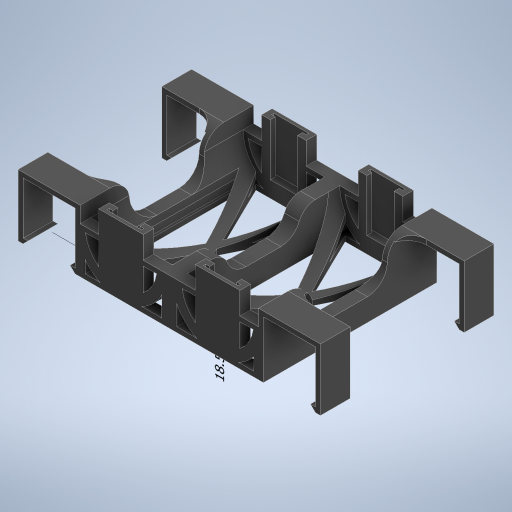
# Autodesk Inventor part: 電池ボックス
Saved by Autodesk Inventor 2024.1 (Build 281209000, 209)
## iProperties
Created: 2024-11-06
Part Number: 電池ボックス
Material: 一般
Document SubType Name: Modeling
Designer: hibik
Density: 1 g/cm^3
Appearance: 既定
Author: hibik
Autodesk Inventor part; units mm, degrees
ref_plane "YZ Plane" through (0, 0, 0) normal (1, 0, 0) x (0, 1, 0)
ref_plane "XZ Plane" through (0, 0, 0) normal (0, 1, 0) x (-1, 0, 0)
ref_plane "XY Plane" through (0, 0, 0) normal (0, 0, 1) x (1, 0, 0)
sketch "スケッチ1" plane through (0, 0, 0) normal (0, 0, 1) x (1, 0, 0)
  line L0 (-59, 0) -> (-38, 0)
  line L1 (-38, 0) -> (-38, -21)
  line L2 (-38, -21) -> (-59, -21)
  line L3 (-59, -21) -> (-59, 0)
  line L4 (-61, 2) -> (-36, 2)
  line L5 (-36, 2) -> (-36, -23)
  line L6 (-36, -23) -> (-61, -23)
  line L7 (-61, -23) -> (-61, 2)
  line L8 (-61, -23) -> (0, -23)
  line L9 (0, -23) -> (0, -21)
  line L10 (0, -21) -> (-61, -21)
  line L11 (-61, -21) -> (-61, -23)
  line L12 (-59, -23) -> (-57, -21)
  line L13 (-38, -23) -> (-40, -21)
  point P0 (0, 0)
  point P1 (-61, -10.5)
  point P2 (-59, -10.5)
  point P3 (-48.5, 2)
  point P4 (-48.5, 0)
  point P5 (-36, -21)
  dimension "d0" = 21
  dimension "d1" = 21
  dimension "d4" = 38
  dimension "d5" = 25
  dimension "d6" = 2
  dimension "d74" = 2
  dimension "d75" = 2
  constraints: 28 end point, 8 point on line, 6 parallel, 4 midpoint, 4 perpendicular, 3 horizontal, 1 horizontal alignment, 1 vertical alignment
  measures "d0" distance of L1.end L2.end
  measures "d1" distance of L0.end L1.end
  measures "d4" distance from line of point (0, 0) L1
  measures "d5" distance of L4.start L4.end
  measures "d6" distance of L8.end L9.end
  measures "d74" distance of L2.end L12.end
  measures "d75" distance from line of L1 L13.end
extrude "押し出し1" add sketch "スケッチ1" along normal blind 70 contours L3 L10 L7 L4 L5 L1 L0 | L2 L12 L6 L7 L10 | L10 L5 L6 L13 L2 | L10 L9 L8 L5
sketch "スケッチ16" plane through (0, 0, 0) normal (0, 0, -1) x (-1, 0, 0)
  circle A0 centre (19.5, -4.5) radius 16.5
  line L0 (0, -21) -> (36, -21) projected
  line L1 (36, -21) -> (36, 2) projected
  line L2 (36, -4.5) -> (0, -4.5)
  line L3 (0, -4.5) -> (0, -21)
  point P0 (0, 0)
  point P1 (19.5, -21)
  point P2 (3, -4.5)
  dimension "d76" = 33
  constraints: 4 end point, 2 horizontal, 1 perpendicular, 1 point on line, 1 vertical, 3 other
extrude "押し出し16" add sketch "スケッチ16" against normal up to surface (70 mm away) contours L1 L0 A0 | A0 L0 L3 L2
sketch "スケッチ17" plane through (-38, -23, 0) normal (0, -1, 0) x (1, 0, 0)
  line L0 (0, 0) -> (38, 0) projected
  line L1 (38, 0) -> (38, 70) projected
  line L2 (0, 70) -> (38, 70) projected
  line L3 (0, 0) -> (0, 70) projected
  line L4 (35, 0) -> (35, 70) projected
  line L5 (0, 65.75) -> (35, 65.75)
  line L6 (35, 65.75) -> (35, 4.25)
  line L7 (35, 4.25) -> (0, 4.25)
  line L8 (0, 4.25) -> (0, 65.75)
  line L9 (9.5, 70) -> (27.5, 70)
  line L10 (27.5, 70) -> (27.5, 65.75)
  line L11 (27.5, 65.75) -> (9.5, 65.75)
  line L12 (9.5, 65.75) -> (9.5, 70)
  line L13 (9.5, 0) -> (27.5, 0)
  line L14 (27.5, 0) -> (27.5, 4.25)
  line L15 (27.5, 4.25) -> (9.5, 4.25)
  line L16 (9.5, 4.25) -> (9.5, 0)
  line L17 (2, 0) -> (2, 70) projected
  point P0 (38, 0)
  point P1 (35, 35)
  point P2 (27.5, 0)
  point P3 (27.5, 70)
  dimension "d79" = 61.5
  dimension "d80" = 18
  dimension "d82" = 7.5
  dimension "d97" = 7.5
  constraints: 24 end point, 6 parallel, 6 point on line, 3 horizontal, 3 perpendicular, 2 collinear, 2 midpoint
  measures "d79" distance between parallel lines of L7 L5
  measures "d80" distance between parallel lines of L10 L12
  measures "d82" distance between parallel lines of L4 L10
  measures "d97" distance between parallel lines of L17 L12
extrude "押し出し17" add sketch "スケッチ17" against normal blind 27.5 contours L16 L7 L14 L0 | L12 L2 L10 L5
sketch "スケッチ18" plane through (-38, 4.5, 0) normal (0, 1, 0) x (1, 0, 0)
  line L0 (11.5, -2.25) -> (25.5, -2.25)
  line L1 (25.5, -2.25) -> (25.5, -1.25)
  line L2 (25.5, -1.25) -> (11.5, -1.25)
  line L3 (11.5, -1.25) -> (11.5, -2.25)
  line L4 (27.5, 0) -> (9.5, 0) projected
  line L5 (9.5, -4.25) -> (27.5, -4.25) projected
  line L6 (13, -2.25) -> (24, -2.25)
  line L7 (24, -2.25) -> (24, -4.25)
  line L8 (24, -4.25) -> (13, -4.25)
  line L9 (13, -4.25) -> (13, -2.25)
  line L10 (60.0191, -35) -> (-21.9972, -35)
  line L11 (9.5, -70) -> (27.5, -70) projected
  line L12 (11.5, -67.75) -> (25.5, -67.75)
  line L13 (25.5, -67.75) -> (25.5, -68.75)
  line L14 (25.5, -68.75) -> (11.5, -68.75)
  line L15 (11.5, -68.75) -> (11.5, -67.75)
  line L16 (27.5, -70) -> (9.5, -70)
  line L17 (9.5, -65.75) -> (27.5, -65.75)
  line L18 (13, -67.75) -> (24, -67.75)
  line L19 (24, -67.75) -> (24, -65.75)
  line L20 (24, -65.75) -> (13, -65.75)
  line L21 (13, -65.75) -> (13, -67.75)
  point P0 (38, 0)
  point P1 (18.5, -1.25)
  point P2 (18.5, 0)
  point P3 (13, -4.25)
  point P4 (24, -2.25)
  point P5 (18.5, -68.75)
  point P6 (18.5, -70)
  dimension "d88" = 14
  dimension "d89" = 1
  dimension "d90" = 2
  dimension "d91" = 1.5
  dimension "d92" = 1.5
  dimension "d95" = 35
  dimension "d96" = 35
  constraints: 38 end point, 12 symmetric about line, 4 parallel, 4 point on line, 3 horizontal, 2 midpoint, 2 perpendicular, 1 vertical alignment
  measures "d88" distance of L2.end L1.end
  measures "d89" distance of L1.end L0.end
  measures "d90" distance between parallel lines of L5 L0
  measures "d91" distance between parallel lines of L3 L9
  measures "d92" distance between parallel lines of L1 L7
  measures "d95" distance between parallel lines of L11 L10
  measures "d96" distance between parallel lines of L4 L10
extrude "押し出し18" cut sketch "スケッチ18" against normal blind 21
sketch "スケッチ19" plane through (-3, -4.5, 0) normal (0, 1, 0) x (1, 0, 0)
  line L0 (-35, -70) -> (3, -70) projected
  line L1 (-7.5, -70) -> (-7.5, -65.75) projected
  line L2 (0, -70) -> (-7.5, -70)
  line L3 (-7.5, -70) -> (-7.5, -65.75)
  line L4 (-7.5, -65.75) -> (0, -65.75)
  line L5 (0, -65.75) -> (0, -70)
  line L6 (-33, -70) -> (-33, 0) projected
  line L7 (-25.5, -70) -> (-33, -70)
  line L8 (-33, -70) -> (-33, -65.75)
  line L9 (-33, -65.75) -> (-25.5, -65.75)
  line L10 (-25.5, -65.75) -> (-25.5, -70)
  line L11 (-25.5, -65.75) -> (-25.5, -70) projected
  line L12 (0, 0) -> (0, -70) projected
  line L13 (-7.5, 0) -> (-7.5, -4.25) projected
  line L14 (-7.5, -4.25) -> (0, -4.25)
  line L15 (0, -4.25) -> (0, 0)
  line L16 (0, 0) -> (-7.5, 0)
  line L17 (-7.5, 0) -> (-7.5, -4.25)
  line L18 (-25.5, -4.25) -> (-33, -4.25)
  line L19 (-33, -4.25) -> (-33, 0)
  line L20 (-33, 0) -> (-25.5, 0)
  line L21 (-25.5, 0) -> (-25.5, -4.25)
  line L22 (-25.5, 0) -> (-25.5, -4.25) projected
  point P0 (3, 0)
  point P1 (0, -4.25)
  constraints: 32 end point, 8 parallel, 5 point on line, 4 horizontal, 4 perpendicular, 3 collinear
extrude "押し出し19" add sketch "スケッチ19" against normal up to surface (18.5 mm away)
sketch "スケッチ20" plane through (0, 0, 70) normal (0, 0, 1) x (1, 0, 0)
  arc A0 (-36, -4.5) -> (-3, -4.5) centre (-19.5, -4.5) ccw projected
  line L0 (-25, -16.5) -> (-14, -16.5) projected
  line L1 (-36, -4.5) -> (-28.5, -4.5) construction
  line L2 (-10.5, -4.5) -> (0, -4.5) construction
  line L3 (-28.5, -4.5) -> (-28.5, 4.5) projected
  line L4 (-28.5, -4.5) -> (-10.5, -4.5) construction
  circle A1 centre (-19.5, -4.5) radius 14.5
  line L5 (-33.8614, -6.5) -> (-28.5, -6.5)
  line L6 (-28.5, -6.5) -> (-28.5, -15.8688)
  line L7 (-5.1386, -6.5) -> (-10.5, -6.5)
  line L8 (-10.5, -6.5) -> (-10.5, -15.8688)
  line L9 (-12.5, 4.5) -> (-26.5, 4.5) projected
  line L10 (-12.5, 4.5) -> (-12.5, -16.5) construction
  line L11 (-12.5, -16.5) -> (-26.5, -16.5) projected
  line L12 (-26.5, 4.5) -> (-26.5, -16.5) construction
  line L13 (-23, 1.5) -> (-16, 1.5)
  line L14 (-16, 1.5) -> (-16, -13.5)
  line L15 (-16, -13.5) -> (-23, -13.5)
  line L16 (-23, -13.5) -> (-23, 1.5)
  line L17 (-14, 4.5) -> (-14, -16.5) construction
  line L18 (-12.5, 4.5) -> (-26.5, 4.5) projected
  circle A2 centre (-19.5, -4.5) radius 18.5
  line L19 (-34, -15.9891) -> (-34, -21)
  line L20 (-34, -21) -> (-27.8666, -21)
  line L21 (-11.1334, -21) -> (-3, -21)
  line L22 (-3, -21) -> (-3, -12.8666)
  line L23 (-38, 0) -> (-38, -21) projected
  line L24 (-38, -21) -> (-40, -21) projected
  line L25 (0, -23) -> (0, -4.5) projected
  line L26 (-36, -4.5) -> (-36, 2) projected
  point P0 (0, 0)
  point P1 (-16, -6)
  point P2 (-14, -6)
  point P3 (-19.5, 1.5)
  point P4 (-19.5, 4.5)
  dimension "d101" = 2
  dimension "d103" = 2
  dimension "d107" = 2
  dimension "d108" = 2
  dimension "d109" = 2
  dimension "d110" = 3
  dimension "d133" = 2
  dimension "d136" = 2
  constraints: 26 end point, 8 point on circle, 5 perpendicular, 4 horizontal, 4 midpoint, 3 point on line, 2 centre point, 2 coincident, 2 collinear, 2 parallel, 1 horizontal alignment, 1 vertical, 1 vertical alignment
  measures "d101" radial gap between concentric circles of A0 A1
  measures "d103" distance between parallel lines of L1 L5
  measures "d107" distance between parallel lines of L12 L6
  measures "d108" distance between parallel lines of L8 L10
  measures "d109" distance between parallel lines of L17 L14
  measures "d110" distance between parallel lines of L9 L13
  measures "d133" radial gap between concentric circles of A0 A2
  measures "d136" distance between parallel lines of L26 L19
extrude "押し出し20" cut sketch "スケッチ20" against normal through all contours L5 L6 A1 | A1 L8 L7 | A2 L20 L19 | A2 L22 L21
sketch "スケッチ22" plane through (-61, 2, 0) normal (0, 1, 0) x (1, 0, 0)
  line L0 (0, -12) -> (23, -12)
  line L1 (23, -12) -> (23, -58)
  line L2 (23, -58) -> (0, -58)
  line L3 (0, -58) -> (0, -12)
  line L4 (23, 0) -> (23, -70) projected
  line L5 (25, 0) -> (0, 0) projected
  line L6 (25, -70) -> (0, -70) projected
  line L7 (0, 0) -> (0, -70) projected
  point P0 (61, 0)
  dimension "d118" = 12
  dimension "d119" = 12
  constraints: 8 end point, 2 collinear, 2 parallel, 1 horizontal, 1 perpendicular
  measures "d118" distance between parallel lines of L5 L0
  measures "d119" distance between parallel lines of L6 L2
extrude "押し出し22" cut sketch "スケッチ22" against normal through all contours L0 L1 L2 L3
fillet "フィレット4" radius 8 2 edges at (-38, 1, 12) (-38, 1, 58)
sketch "スケッチ23" plane through (-38, -23, 0) normal (0, -1, 0) x (1, 0, 0)
  line L0 (35, 4.25) -> (2, 4.25) projected
  line L1 (2, 65.75) -> (2, 4.25) projected
  line L2 (2, 65.75) -> (35, 65.75) projected
  line L3 (35, 4.25) -> (35, 65.75) projected
  line L4 (5, 65.75) -> (5, 4.25)
  line L5 (6.7975, 66.6268) -> (36.7975, 5.1268)
  line L6 (36.7975, 5.1268) -> (33.2025, 3.3732)
  line L7 (33.2025, 3.3732) -> (3.2025, 64.8732)
  line L8 (3.2025, 64.8732) -> (6.7975, 66.6268)
  line L9 (6.7975, 66.6268) -> (33.2025, 3.3732) construction
  line L10 (36.7975, 5.1268) -> (3.2025, 64.8732) construction
  line L11 (3.2025, 5.1268) -> (33.2025, 66.6268)
  line L12 (33.2025, 66.6268) -> (36.7975, 64.8732)
  line L13 (36.7975, 64.8732) -> (6.7975, 3.3732)
  line L14 (6.7975, 3.3732) -> (3.2025, 5.1268)
  line L15 (3.2025, 5.1268) -> (36.7975, 64.8732) construction
  line L16 (33.2025, 66.6268) -> (6.7975, 3.3732) construction
  point P0 (38, 0)
  point P1 (20, 35)
  point P2 (20, 35)
  point P3 (5, 8.8118)
  point P4 (17.7747, 35)
  point P5 (5, 61.1882)
  point P6 (20, 30.4382)
  point P7 (7.2253, 4.25)
  point P8 (32.7747, 4.25)
  point P9 (35, 61.1882)
  point P10 (22.2253, 35)
  point P11 (35, 8.8118)
  point P12 (20, 39.5618)
  point P13 (32.7747, 65.75)
  point P14 (7.2253, 65.75)
  dimension "d123" = 3
  dimension "d124" = 4
  constraints: 26 end point, 8 midpoint, 4 parallel, 3 perpendicular, 2 point on line, 1 equal length
  measures "d123" distance between parallel lines of L1 L4
  measures "d124" distance between parallel lines of L13 L11
extrude "押し出し23" cut sketch "スケッチ23" against normal through all contours L13 L7 L0 | L4 L7 L11 | L13 L3 L5 | L5 L2 L11
sketch "スケッチ25" plane through (-38, -21, 0) normal (-1, 0, 0) x (0, 0, 1)
  line L0 (61.1882, 7.0132) -> (8.8118, 7.0132) projected
  line L1 (12, -2) -> (12, 23) projected
  line L2 (0, 23) -> (12, 23) projected
  line L3 (0, 23) -> (0, -2) projected
  line L4 (0, -2) -> (12, -2) projected
  line L5 (58, 23) -> (58, -2) projected
  line L6 (58, -2) -> (70, -2) projected
  line L7 (70, 23) -> (70, -2) projected
  line L8 (58, 23) -> (70, 23) projected
  line L9 (0, 23) -> (70, 23) projected
  line L10 (20, 7.0132) -> (50, 7.0132)
  line L11 (50, 7.0132) -> (50, 23)
  line L12 (50, 23) -> (20, 23)
  line L13 (20, 23) -> (20, 7.0132)
  line L14 (20, 21) -> (20, 23) projected
  line L15 (50, 23) -> (50, 21) projected
  point P0 (0, 21)
  point P1 (20, 23)
  point P2 (50, 7.0132)
  constraints: 8 end point, 2 collinear, 2 parallel, 2 point on line, 1 horizontal, 1 perpendicular
extrude "押し出し24" cut sketch "スケッチ25" against normal through all contours L0 L13 L9 L11
fillet "フィレット5" radius 8 6 edges at (-37, 2, 50) (-37, 2, 20) (-35.5, -13.9868, 50) (-35.5, -13.9868, 20) (-1.5, -13.9868, 20) (-1.5, -13.9868, 50)
fillet "フィレット6" radius 7 2 edges at (-1.5, -4.5, 50) (-1.5, -4.5, 20)
mirror "ミラー4" about plane through (0, -23, 0) normal (1, 0, 0)
sketch "スケッチ26" plane through (0, 0, 70) normal (0, 0, 1) x (1, 0, 0)
  line L0 (40, -21) -> (38, -23) projected
  line L1 (38, -21) -> (40, -21) projected
  line L2 (38, -21) -> (38, -23)
  line L3 (38, -21) -> (38, -23) projected
  point P0 (0, 0)
  constraints: 2 end point, 1 collinear, 1 point on line
extrude "押し出し25" cut sketch "スケッチ26" against normal through all
equation "\"d0\" = d1"
equation "\"d75\" = d74"
equation "\"d97\" = d82"
equation "\"d92\" = d91"
equation "\"d95\" = d96"
equation "\"d103\" = d101"
equation "\"d107\" = d101"
equation "\"d108\" = d107"
equation "\"d109\" = d101"
equation "\"d119\" = d118"
